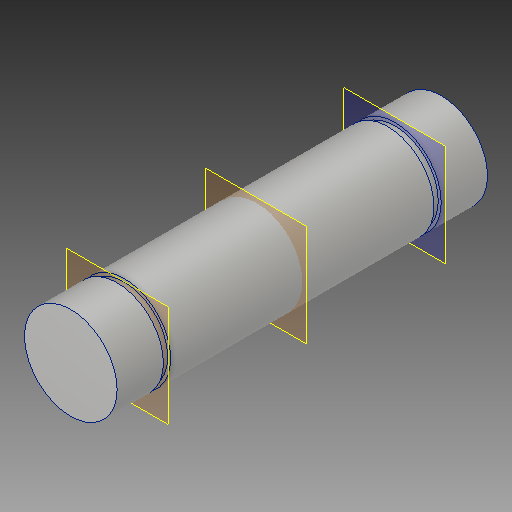
# Autodesk Inventor part: Linear Actuator Top Pin .5in. Dia.
Saved by Autodesk Inventor 2019 (Build 230136000, 136)
## iProperties
Created: 2018-10-30
Part Number: Linear Actuator Top Pin .5in. Dia.
Material: Aluminum 6061
Document SubType Name: Modeling
Designer: Alex Barnett
Density: 2.7 g/cm^3
Appearance: Aluminum - Flat
Mass: 17.291 g
Surface Area: 23.3791 cm^2
Volume: 6.40409 cm^3
Author: Alex Barnett
Autodesk Inventor part; units mm, degrees
ref_plane "YZ Plane" through (0, 0, 0) normal (1, 0, 0) x (0, 1, 0)
ref_plane "XZ Plane" through (0, 0, 0) normal (0, 1, 0) x (-1, 0, 0)
sketch "Sketch1" plane through (0, 0, 0) normal (0, 0, 1) x (1, 0, 0)
  circle A0 centre (0, 0) radius 6.35
  dimension "d0" = 12.7
  constraints: 1 centre point, 1 coincident
  measures "d0" diameter of A0
extrude "Extrusion1" add sketch "Sketch1" along normal mid plane 50.8
ref_plane "Work Plane1" through (0, 0, 19.05) normal (0, 0, 1) x (1, 0, 0)
sketch "Sketch2" plane through (0, 0, 19.05) normal (0, 0, 1) x (1, 0, 0)
  circle A0 centre (0, 0) radius 6.35 projected
  circle A1 centre (0, 0) radius 6.35
  circle A2 centre (0, 0) radius 5.9436
  dimension "d4" = 12.7
  dimension "d5" = 11.8872
  constraints: 2 centre point, 2 coincident
  measures "d4" diameter of A1
  measures "d5" diameter of A2
extrude "Extrusion2" cut sketch "Sketch2" against normal blind 0.9906
mirror "Mirror1" about plane through (0, 0, 0) normal (0, 0, 1) of "Extrusion2"
ref_plane "Work Plane2" through (0, 0, -19.05) normal (0, 0, 1) x (1, 0, 0)
body "Solid1"
